Autodesk Fusion 360 part; units mm, degrees
(part 2 of 2)
sketch "Sketch7" plane through (0, -85, 0) normal (0, -1, 0) x (1, 0, 0)
  line L0 (-105, 15) -> (0, 15)
  line L1 (0, 15) -> (0, 90)
  line L2 (0, 90) -> (-120, 90)
  line L3 (-120, 90) -> (-120, 72)
  line L4 (-120, 72) -> (-105, 72)
  line L5 (-105, 72) -> (-105, 15)
  circle A0 centre (-135, -8) radius 75
  dimension "d159" = 150
  dimension "d160" = 80
  dimension "d161" = 30
  measures "d159" diameter of A0
  measures "d160" distance of L4 A0.centre
  measures "d161" distance of L5 A0.centre
extrude "Extrude10" cut sketch "Sketch7" against normal blind 10 contours L0 L5 A0 | L0 L5 A0 bodies 1
sketch "Sketch8" plane through (0, 85, 0) normal (0, 1, 0) x (-1, 0, 0)
  line L0 (0, 15) -> (105, 15)
  line L1 (105, 15) -> (105, 72)
  line L2 (105, 72) -> (120, 72)
  line L3 (120, 72) -> (120, 90)
  line L4 (120, 90) -> (0, 90)
  line L5 (0, 90) -> (0, 15)
  circle A0 centre (135, -8) radius 75
  dimension "d164" = 150
  dimension "d165" = 30
  dimension "d166" = 80
  measures "d164" diameter of A0
  measures "d165" distance of L1 A0.centre
  measures "d166" distance of L2 A0.centre
extrude "Extrude11" cut sketch "Sketch8" against normal blind 10 contours L0 L1 A0 | L0 L1 A0 bodies 1
sketch "Sketch9" plane through (0, 75, 0) normal (0, -1, 0) x (1, 0, 0)
  arc A0 (-62.192, 10) -> (-105, 60.7386) centre (-135, -8) ccw
  line L0 (-62.192, 10) -> (0, 10)
  line L1 (0, 10) -> (0, 85)
  line L2 (0, 85) -> (-115, 85)
  line L3 (-115, 85) -> (-115, 72)
  line L4 (-115, 72) -> (-105, 72)
  line L5 (-105, 72) -> (-105, 60.7386)
  line L6 (-100, 80) -> (-5, 80)
  line L7 (-5, 80) -> (-5, 15)
  line L8 (-5, 15) -> (-100, 15)
  line L9 (-100, 15) -> (-100, 80)
  dimension "d199" = 95
  dimension "d200" = 65
  dimension "d201" = 5
  dimension "d202" = 5
  constraint horizontal L6
  constraint vertical L7
  constraint horizontal L8
  constraint vertical L9
  measures "d199" distance of L6.start L6.end
  measures "d200" distance of L6.end L7.end
  measures "d201" distance of L1 L7
  measures "d202" distance of L2 L6
extrude "Extrude12" cut sketch "Sketch9" against normal blind 5 contours A0 L6 L7 L8 L9 bodies 1
sketch "Sketch10" plane through (0, -75, 0) normal (0, 1, 0) x (-1, 0, 0)
  arc A0 (105, 60.7386) -> (62.192, 10) centre (135, -8) ccw
  line L0 (105, 60.7386) -> (105, 72)
  line L1 (105, 72) -> (115, 72)
  line L2 (115, 72) -> (115, 85)
  line L3 (115, 85) -> (0, 85)
  line L4 (0, 85) -> (0, 10)
  line L5 (0, 10) -> (62.192, 10)
  line L6 (100, 80) -> (5, 80)
  line L7 (5, 80) -> (5, 15)
  line L8 (5, 15) -> (100, 15)
  line L9 (100, 15) -> (100, 80)
  dimension "d203" = 65
  dimension "d204" = 95
  dimension "d205" = 5
  dimension "d206" = 5
  constraint horizontal L6
  constraint vertical L7
  constraint horizontal L8
  constraint vertical L9
  measures "d203" distance of L6 L8
  measures "d204" distance of L7 L9
  measures "d205" distance of L3 L6
  measures "d206" distance of L4 L7
extrude "Extrude13" cut sketch "Sketch10" against normal blind 5 contours A0 L6 L7 L8 L9 bodies 1
sketch "Sketch11" plane through (0, 0, 10) normal (0, 0, 1) x (-1, 0, 0)
  line L0 (0, 75) -> (0, -75)
  line L1 (0, -75) -> (62.192, -75)
  line L2 (62.192, -75) -> (105, -75)
  line L3 (105, -75) -> (105, -20)
  arc A0 (110, -15) -> (105, -20) centre (110, -20) ccw
  line L4 (110, -15) -> (115, -15)
  line L5 (115, -15) -> (115, 15)
  line L6 (115, 15) -> (110, 15)
  arc A1 (105, 20) -> (110, 15) centre (110, 20) ccw
  line L7 (105, 20) -> (105, 75)
  line L8 (105, 75) -> (62.192, 75)
  line L9 (62.192, 75) -> (0, 75)
  line L10 (10, 70) -> (60, 70)
  line L11 (60, 70) -> (60, -70)
  line L12 (60, -70) -> (10, -70)
  line L13 (10, -70) -> (10, 70)
  line L14 (60, 5) -> (110, 5)
  line L15 (110, 5) -> (110, -5)
  line L16 (110, -5) -> (60, -5)
  line L17 (60, -5) -> (60, 5)
  line L18 (60, -5) -> (10, -5)
  line L19 (10, -5) -> (10, 5)
  line L20 (10, 5) -> (60, 5)
  line L21 (60, 5) -> (60, -5)
  dimension "d207" = 50
  dimension "d208" = 140
  dimension "d209" = 10
  dimension "d210" = 5
  dimension "d211" = 50
  dimension "d212" = 10
  dimension "d213" = 70
  constraint horizontal L10
  constraint vertical L11
  constraint horizontal L12
  constraint vertical L13
  constraint horizontal L14
  constraint vertical L15
  constraint horizontal L16
  constraint vertical L17
  constraint coincident L11 L14.start
  constraint horizontal L18
  constraint vertical L19
  constraint horizontal L20
  constraint vertical L21
  constraint collinear L14 L20
  constraint collinear L13 L19
  measures "d207" distance of L10.start L10.end
  measures "d208" distance of L10.start L12.end
  measures "d209" distance of L0 L13
  measures "d210" distance of L9 L10
  measures "d211" distance of L14.start L14.end
  measures "d212" distance of L14.end L15.end
  measures "d213" distance of L8 L14
extrude "Extrude14" cut sketch "Sketch11" against normal blind 5 contours L10 L11 L13 L20 | L11 L12 L13 L18 bodies 1
sketch "Sketch12" plane through (-115, 0, 0) normal (1, 0, 0) x (0, 1, 0)
  line L0 (75, 85) -> (-75, 85)
  line L1 (-75, 85) -> (-75, 72)
  line L2 (-75, 72) -> (-15, 72)
  line L3 (-15, 72) -> (-15, 10)
  line L4 (-15, 10) -> (15, 10)
  line L5 (15, 10) -> (15, 72)
  line L6 (15, 72) -> (75, 72)
  line L7 (75, 72) -> (75, 85)
  line L8 (-73, 83) -> (73, 83)
  line L9 (73, 83) -> (73, 74)
  line L10 (73, 74) -> (-73, 74)
  line L11 (-73, 74) -> (-73, 83)
  line L12 (-12, 74) -> (12, 74)
  line L13 (12, 74) -> (12, 12)
  line L14 (12, 12) -> (-12, 12)
  line L15 (-12, 12) -> (-12, 74)
  line L16 (-5, 83) -> (5, 83)
  line L17 (5, 83) -> (5, 12)
  line L18 (5, 12) -> (-5, 12)
  line L19 (-5, 12) -> (-5, 83)
  dimension "d214" = 2
  dimension "d215" = 146
  dimension "d216" = 9
  dimension "d217" = 2
  dimension "d218" = 62
  dimension "d219" = 24
  dimension "d220" = 3
  dimension "d239" = 10
  constraint horizontal L8
  constraint vertical L9
  constraint horizontal L10
  constraint vertical L11
  constraint horizontal L12
  constraint vertical L13
  constraint horizontal L14
  constraint vertical L15
  constraint coincident L10 L12.start
  constraint horizontal L16
  constraint vertical L17
  constraint horizontal L18
  constraint vertical L19
  constraint coincident L14 L17.end
  constraint coincident L8 L16.start
  constraint midpoint L8 L16
  measures "d214" distance of L0 L8
  measures "d215" distance of L9.end L10.end
  measures "d216" distance of L8.start L10.end
  measures "d217" distance of L1 L11
  measures "d218" distance of L12.end L13.end
  measures "d219" distance of L13.end L14.end
  measures "d220" distance of L5 L13
  measures "d239" distance of L17 L19
extrude "Extrude15" cut sketch "Sketch12" against normal blind 5 contours L8 L10 L11 L12 L19 | L8 L9 L10 L12 L17 | L10 L12 L14 L15 L19 | L10 L12 L13 L14 L17 bodies 1
sketch "Sketch13" plane through (0, -63, 0) normal (0, 1, 0) x (-1, 0, 0)
  line L0 (96, 32.5) -> (78, 32.5)
  line L1 (78, 32.5) -> (78, 11)
  line L2 (78, 11) -> (96, 11)
  line L3 (96, 11) -> (96, 32.5)
  line L4 (94, 31) -> (80, 31)
  line L5 (80, 31) -> (80, 13)
  line L6 (80, 13) -> (94, 13)
  line L7 (94, 13) -> (94, 31)
  line L8 (89.5, 19.5) -> (84.5, 19.5)
  line L9 (84.5, 19.5) -> (84.5, 24.5)
  line L10 (84.5, 24.5) -> (89.5, 24.5)
  line L11 (89.5, 24.5) -> (89.5, 19.5)
  line L12 (89.5, 19.5) -> (84.5, 24.5) construction
  line L13 (84.5, 19.5) -> (89.5, 24.5) construction
  point P0 (87, 22)
  dimension "d183" = 1.5
  dimension "d184" = 2
  dimension "d185" = 18
  dimension "d186" = 14
  dimension "d187" = 5
  dimension "d188" = 5
  dimension "d189" = 9
  dimension "d190" = 7
  constraint horizontal L4
  constraint vertical L5
  constraint horizontal L6
  constraint vertical L7
  constraint horizontal L8
  constraint perpendicular L8 L9
  constraint parallel L8 L10
  constraint parallel L9 L11
  constraint coincident L12 P0
  constraint coincident L13 P0
  measures "d183" distance of L0 L4
  measures "d184" distance of L3 L7
  measures "d185" distance of L4 L6
  measures "d186" distance of L5 L7
  measures "d187" distance of L9.end L10.end
  measures "d188" distance of L8.end L9.end
  measures "d189" distance of L4 P0
  measures "d190" distance of L7 P0
extrude "Extrude4'" cut sketch "Sketch13" against normal blind 5 contours L4 L5 L6 L7 sketch seen with x (0, 1, 0) y (-1, 0, 0) z (0, 0, 1) at (-43, 100.7041, -11) bodies 5 in component "rest_casing v2 (1)"
sketch "Sketch14" plane through (0, -23, 0) normal (0, -1, 0) x (1, 0, 0)
  line L0 (-76, 32.5) -> (-96, 32.5)
  line L1 (-96, 32.5) -> (-96, 11)
  line L2 (-96, 11) -> (-76, 11)
  line L3 (-76, 11) -> (-76, 32.5)
  line L4 (-94, 31) -> (-78, 31)
  line L5 (-78, 31) -> (-78, 12)
  line L6 (-78, 12) -> (-94, 12)
  line L7 (-94, 12) -> (-94, 31)
  line L8 (-83.5, 19) -> (-88.5, 19)
  line L9 (-88.5, 19) -> (-88.5, 24)
  line L10 (-88.5, 24) -> (-83.5, 24)
  line L11 (-83.5, 24) -> (-83.5, 19)
  line L12 (-83.5, 19) -> (-88.5, 24) construction
  line L13 (-88.5, 19) -> (-83.5, 24) construction
  point P0 (-86, 21.5)
  dimension "d191" = 1.5
  dimension "d192" = 2
  dimension "d193" = 19
  dimension "d194" = 16
  dimension "d195" = 5
  dimension "d196" = 5
  dimension "d197" = 9.5
  dimension "d198" = 8
  constraint horizontal L4
  constraint vertical L5
  constraint horizontal L6
  constraint vertical L7
  constraint horizontal L8
  constraint perpendicular L8 L9
  constraint parallel L8 L10
  constraint parallel L9 L11
  constraint coincident L12 P0
  constraint coincident L13 P0
  measures "d191" distance of L0 L4
  measures "d192" distance of L1 L7
  measures "d193" distance of L4 L6
  measures "d194" distance of L5 L7
  measures "d195" distance of L9.end L10.end
  measures "d196" distance of L8.end L9.end
  measures "d197" distance of L4 P0
  measures "d198" distance of L7 P0
extrude "Extrude5'" cut sketch "Sketch14" against normal blind 5 contours L4 L5 L6 L7 sketch seen with x (0, 1, 0) y (-1, 0, 0) z (0, 0, 1) at (-43, 100.7041, -11) bodies 5 in component "rest_casing v2 (1)"
sketch "Sketch15" plane through (0, 23, 0) normal (0, 1, 0) x (-1, 0, 0)
  line L0 (96, 32.5) -> (78, 32.5)
  line L1 (78, 32.5) -> (78, 11)
  line L2 (78, 11) -> (96, 11)
  line L3 (96, 11) -> (96, 32.5)
  line L4 (80, 31) -> (94, 31)
  line L5 (94, 31) -> (94, 12)
  line L6 (94, 12) -> (80, 12)
  line L7 (80, 12) -> (80, 31)
  line L8 (89.5, 19) -> (84.5, 19)
  line L9 (84.5, 19) -> (84.5, 24)
  line L10 (84.5, 24) -> (89.5, 24)
  line L11 (89.5, 24) -> (89.5, 19)
  line L12 (89.5, 19) -> (84.5, 24) construction
  line L13 (84.5, 19) -> (89.5, 24) construction
  point P0 (87, 21.5)
  dimension "d221" = 19
  dimension "d222" = 14
  dimension "d223" = 1.5
  dimension "d224" = 2
  dimension "d225" = 5
  dimension "d226" = 5
  dimension "d227" = 9.5
  dimension "d228" = 7
  constraint horizontal L4
  constraint vertical L5
  constraint horizontal L6
  constraint vertical L7
  constraint horizontal L8
  constraint perpendicular L8 L9
  constraint parallel L8 L10
  constraint parallel L9 L11
  constraint coincident L12 P0
  constraint coincident L13 P0
  measures "d221" distance of L4.end L5.end
  measures "d222" distance of L4.start L4.end
  measures "d223" distance of L0 L4
  measures "d224" distance of L3 L5
  measures "d225" distance of L9.end L10.end
  measures "d226" distance of L8.end L9.end
  measures "d227" distance of L4 P0
  measures "d228" distance of L5 P0
extrude "Extrude4''" cut sketch "Sketch15" against normal blind 5 contours L4 L5 L6 L7 sketch seen with x (0, 1, 0) y (-1, 0, 0) z (0, 0, 1) at (43, 100.7041, -11) bodies 3 in component "rest_casing v2"
sketch "Sketch16" plane through (0, 63, 0) normal (0, -1, 0) x (1, 0, 0)
  line L0 (-76, 32.5) -> (-96, 32.5)
  line L1 (-96, 32.5) -> (-96, 11)
  line L2 (-96, 11) -> (-76, 11)
  line L3 (-76, 11) -> (-76, 32.5)
  line L4 (-94, 31) -> (-78, 31)
  line L5 (-78, 31) -> (-78, 12)
  line L6 (-78, 12) -> (-94, 12)
  line L7 (-94, 12) -> (-94, 31)
  line L8 (-83.5, 19) -> (-88.5, 19)
  line L9 (-88.5, 19) -> (-88.5, 24)
  line L10 (-88.5, 24) -> (-83.5, 24)
  line L11 (-83.5, 24) -> (-83.5, 19)
  line L12 (-83.5, 19) -> (-88.5, 24) construction
  line L13 (-88.5, 19) -> (-83.5, 24) construction
  point P0 (-86, 21.5)
  dimension "d229" = 16
  dimension "d230" = 19
  dimension "d231" = 2
  dimension "d232" = 1.5
  dimension "d233" = 5
  dimension "d234" = 5
  dimension "d235" = 7
  dimension "d236" = 8
  constraint horizontal L4
  constraint vertical L5
  constraint horizontal L6
  constraint vertical L7
  constraint horizontal L8
  constraint perpendicular L8 L9
  constraint parallel L8 L10
  constraint parallel L9 L11
  constraint coincident L12 P0
  constraint coincident L13 P0
  measures "d229" distance of L4.start L4.end
  measures "d230" distance of L4.end L5.end
  measures "d231" distance of L3 L5
  measures "d232" distance of L0 L4
  measures "d233" distance of L9.end L10.end
  measures "d234" distance of L8.end L9.end
  measures "d235" distance of L4 L10
  measures "d236" distance of L5 P0
extrude "Extrude5''" cut sketch "Sketch16" against normal blind 5 contours L4 L5 L6 L7 sketch seen with x (0, 1, 0) y (-1, 0, 0) z (0, 0, 1) at (43, 100.7041, -11) bodies 3 in component "rest_casing v2"
split "Split2" by plane through (0, 0, 0) normal (0, 1, 0) bodies 1 makes body 11 at (-35, 30, 0)
component "rest_casing v2" placed x (0, -1, 0) y (1, 0, 0) z (0, 0, 1) at (-100.7041, 43, 11)
component "rest_casing v2 (1)" placed x (0, -1, 0) y (1, 0, 0) z (0, 0, 1) at (-100.7041, -43, 11)
equation "d133 = 170 mm - 10 mm"
